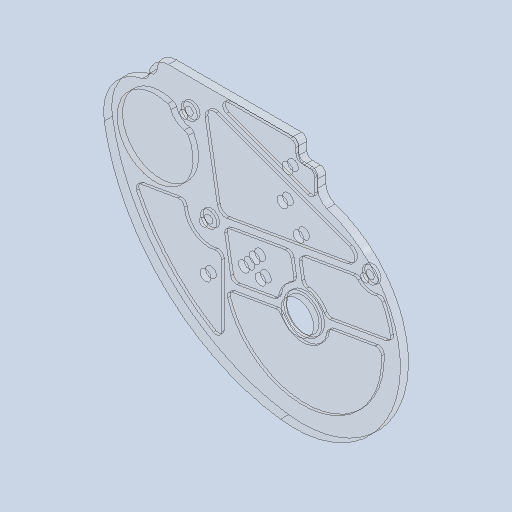
# Autodesk Inventor part: 足外フレーム
Saved by Autodesk Inventor 2023 (Build 270158000, 158)
## iProperties
Created: 2022-01-10
Part Number: 足外フレーム
Material: Polycarbonate, Clear
Document SubType Name: Modeling
Designer: acps
Density: 1.2 g/cm^3
Appearance: Polycarbonate - Clear
Author: acps
Autodesk Inventor part; units mm, degrees
ref_plane "YZ Plane" through (0, 0, 0) normal (1, 0, 0) x (0, 1, 0)
ref_plane "XZ Plane" through (0, 0, 0) normal (0, 1, 0) x (-1, 0, 0)
ref_plane "XY Plane" through (0, 0, 0) normal (0, 0, 1) x (1, 0, 0)
sketch "Sketch6" plane through (0, 0, 0) normal (0, 0, 1) x (1, 0, 0)
  circle A0 centre (46.616, 30) radius 14 construction
  circle A1 centre (67.0906, 21) radius 20.5 construction
  circle A2 centre (100, 0) radius 30 construction
  arc A3 (42.888, 47.6097) -> (28.8684, 26.9964) centre (46.616, 30) ccw
  arc A4 (93.8028, -35.6609) -> (110.9454, 40.1044) centre (98.9344, 3) ccw
  arc A5 (28.8684, 26.9964) -> (93.8028, -35.6609) centre (103.8028, 39.6783) ccw
  line L0 (-13.9923, -60) -> (152.4896, -60) construction
  arc A6 (131.1289, 13.9322) -> (113.2981, 33.8169) centre (98.9344, 3) ccw construction
  circle A7 centre (124.8574, 25) radius 3
  circle A8 centre (58.1571, 43.8132) radius 3
  circle A9 centre (65.359, 13) radius 3
  circle A10 centre (58.1571, 43.8132) radius 4 construction
  arc A11 (42.888, 47.6097) -> (45.3636, 50.3845) centre (42.2376, 50.6816) ccw
  arc A12 (52.4852, 56.8614) -> (45.3636, 50.3845) centre (52.4852, 49.7076) ccw
  line L1 (78.7064, -36) -> (126.3698, -36) construction
  circle A13 centre (58.1571, 43.8132) radius 1.5
  circle A14 centre (65.359, 13) radius 1.5
  circle A15 centre (100, 0) radius 6.025
  circle A16 centre (124.8574, 25) radius 1.5
  arc A17 (68.0566, 48.172) -> (64.0683, 44.8413) centre (67.024, 45.3553) ccw
  line L2 (64.0683, 44.8413) -> (68.5525, 19.0577)
  arc A18 (68.5525, 19.0577) -> (72.0221, 16.6161) centre (71.5081, 19.5718) ccw
  arc A19 (116.6805, 24.3829) -> (117.1992, 30.1552) centre (116.1665, 27.3385) ccw
  line L3 (72.0221, 16.6161) -> (116.6805, 24.3829)
  circle A20 centre (124.8574, 25) radius 6 construction
  circle A21 centre (58.1571, 43.8132) radius 6 construction
  circle A22 centre (65.359, 13) radius 6 construction
  line L4 (68.0566, 48.172) -> (117.1992, 30.1552)
  line L5 (72.9191, 13.7271) -> (93.4394, 17.2959)
  arc A23 (95.7525, 15.6682) -> (93.4394, 17.2959) centre (93.7821, 15.3255) ccw
  line L6 (95.7525, 15.6682) -> (96.7308, 10.0431)
  arc A24 (95.7109, 7.9407) -> (96.7308, 10.0431) centre (94.7604, 9.7004) ccw
  arc A25 (95.7109, 7.9407) -> (91.0775, 1.3563) centre (100, 0) ccw
  arc A26 (89.4429, -0.3135) -> (91.0775, 1.3563) centre (89.1002, 1.6569) ccw
  line L7 (75.7744, -2.6907) -> (89.4429, -0.3135)
  line L8 (100, 0) -> (96.3736, 20.8512) construction
  arc A27 (72.9191, 13.7271) -> (71.2914, 11.414) centre (73.2618, 11.7567) ccw
  line L9 (71.2914, 11.414) -> (73.4613, -1.063)
  arc A28 (73.4613, -1.063) -> (75.7744, -2.6907) centre (75.4317, -0.7203) ccw
  line L10 (129.5563, 5.1403) -> (73.9605, -4.5287) construction
  arc A29 (100.3359, 18.4953) -> (98.7082, 16.1822) centre (100.6786, 16.5249) ccw
  line L11 (98.7082, 16.1822) -> (99.6865, 10.5571)
  arc A30 (99.6865, 10.5571) -> (101.3563, 8.9225) centre (101.6569, 10.8998) ccw
  line L12 (100.3359, 18.4953) -> (118.5316, 21.6598)
  arc A31 (120.3701, 21.017) -> (118.5316, 21.6598) centre (118.8743, 19.6894) ccw
  arc A32 (107.9407, 4.2891) -> (101.3563, 8.9225) centre (100, 0) ccw
  arc A33 (107.9407, 4.2891) -> (110.0431, 3.2692) centre (109.7004, 5.2396) ccw
  line L13 (110.0431, 3.2692) -> (130.7399, 6.8687)
  arc A34 (130.7399, 6.8687) -> (132.3636, 9.204) centre (130.3972, 8.8391) ccw
  arc A35 (120.3701, 21.017) -> (126.8308, 19.3338) centre (124.8574, 25) ccw
  arc A36 (129.2732, 18.3479) -> (126.8308, 19.3338) centre (127.4886, 17.4451) ccw
  arc A37 (132.3636, 9.204) -> (129.2732, 18.3479) centre (98.9344, 3) ccw
  arc A38 (92.0593, -4.2891) -> (108.9225, -1.3563) centre (100, 0) ccw
  arc A39 (92.0593, -4.2891) -> (89.9569, -3.2692) centre (90.2996, -5.2396) ccw
  arc A40 (110.5571, 0.3135) -> (108.9225, -1.3563) centre (110.8998, -1.6569) ccw
  line L14 (110.5571, 0.3135) -> (126.6581, 3.1137)
  line L15 (89.9569, -3.2692) -> (73.8559, -6.0694)
  arc A41 (73.8559, -6.0694) -> (72.2892, -8.6348) centre (74.1986, -8.0398) ccw
  arc A42 (128.999, 1.2279) -> (126.6581, 3.1137) centre (127.0008, 1.1433) ccw
  arc A43 (72.2892, -8.6348) -> (128.999, 1.2279) centre (100, 0) ccw
  arc A44 (51.2056, 43.2263) -> (58.8155, 36.8682) centre (46.616, 30) ccw
  arc A45 (52.4518, 41.9559) -> (51.2056, 43.2263) centre (50.55, 41.3368) ccw
  arc A46 (58.8155, 36.8682) -> (57.3438, 37.8686) centre (57.0728, 35.887) ccw
  arc A47 (52.4518, 41.9559) -> (57.3438, 37.8686) centre (58.1571, 43.8132) ccw
  arc A48 (38.758, 8.8048) -> (67.0654, -22.2439) centre (103.8028, 39.6783) ccw
  arc A49 (40.2222, 11.6328) -> (38.758, 8.8048) centre (40.5648, 9.6624) ccw
  line L16 (40.2222, 11.6328) -> (54.0558, 14.0387)
  arc A50 (56.3913, 12.2377) -> (54.0558, 14.0387) centre (54.3985, 12.0683) ccw
  arc A51 (56.3913, 12.2377) -> (67.5901, 4.2809) centre (65.359, 13) ccw
  arc A52 (70.0859, 2.3434) -> (67.5901, 4.2809) centre (68.0859, 2.3434) ccw
  line L17 (70.0859, 2.3434) -> (70.0859, -20.5239)
  arc A53 (67.0654, -22.2439) -> (70.0859, -20.5239) centre (68.0859, -20.5239) ccw
  arc A54 (34.4673, 18.1085) -> (59.1679, 18.5348) centre (46.616, 30) ccw construction
  line L18 (52.4852, 56.8614) -> (98.4852, 56.8614)
  arc A55 (100.4852, 54.8614) -> (98.4852, 56.8614) centre (98.4852, 54.8614) ccw
  line L19 (100.4852, 54.8614) -> (100.4852, 51.8614)
  arc A56 (100.4852, 51.8614) -> (102.4852, 49.8614) centre (102.4852, 51.8614) ccw
  line L20 (102.4852, 49.8614) -> (105.4852, 49.8614)
  arc A57 (107.4852, 47.8614) -> (105.4852, 49.8614) centre (105.4852, 47.8614) ccw
  line L21 (107.4852, 47.8614) -> (107.4852, 44.8614)
  arc A58 (107.4852, 44.8614) -> (110.9454, 40.1044) centre (112.4852, 44.8614) ccw
  line L22 (71.8306, 49.9836) -> (101.7968, 38.9973)
  arc A59 (72.5191, 53.8614) -> (71.8306, 49.9836) centre (72.5191, 51.8614) ccw
  line L23 (72.5191, 53.8614) -> (95.4852, 53.8614)
  arc A60 (97.4852, 51.8614) -> (95.4852, 53.8614) centre (95.4852, 51.8614) ccw
  line L24 (97.4852, 51.8614) -> (97.4852, 49.8614)
  arc A61 (97.4852, 49.8614) -> (99.4852, 47.8614) centre (99.4852, 49.8614) ccw
  line L25 (99.4852, 47.8614) -> (102.4852, 47.8614)
  arc A62 (104.4852, 45.8614) -> (102.4852, 47.8614) centre (102.4852, 45.8614) ccw
  line L26 (104.4852, 45.8614) -> (104.4852, 40.8751)
  arc A63 (101.7968, 38.9973) -> (104.4852, 40.8751) centre (102.4852, 40.8751) ccw
  circle A64 centre (100, 0) radius 7.025
  circle A65 centre (84.2988, 11.1193) radius 3 construction
  circle A66 centre (80.3175, 6.3665) radius 3 construction
  circle A67 centre (86.4242, 5.295) radius 3 construction
  circle A68 centre (94.5653, 34.0473) radius 3.525 construction
  circle A69 centre (100.4873, 25.9894) radius 2.85 construction
  circle A70 centre (84.2988, 11.1193) radius 2
  circle A71 centre (80.3175, 6.3665) radius 2
  circle A72 centre (86.4242, 5.295) radius 2
  circle A73 centre (94.5653, 34.0473) radius 2
  circle A74 centre (100.4873, 25.9894) radius 2
  circle A75 centre (66.1789, -3.483) radius 3 construction
  circle A76 centre (66.1789, -3.483) radius 2
  circle A77 centre (96.3994, 45.7756) radius 1.25 construction
  circle A78 centre (96.3994, 45.7756) radius 2
  point P0 (0, 0)
  point P1 (100, 0)
  point P2 (44.5807, 48.5912)
  point P3 (47.672, 55)
  point P4 (132.0393, 7.6974)
  dimension "d196" = 4
  dimension "d197" = 60
  dimension "d198" = 76
  dimension "d199" = 39
  dimension "d200" = 5
  dimension "d201" = 6
  dimension "d202" = 6
  dimension "d203" = 25
  dimension "d204" = 6
  dimension "d205" = 37
  dimension "d206" = 13
  dimension "d207" = 1
  dimension "d208" = 3.14
  dimension "d209" = 48.5912
  dimension "d210" = 42.888
  dimension "d211" = 24
  dimension "d212" = 3
  dimension "d213" = 3
  dimension "d214" = 12.05
  dimension "d215" = 3
  dimension "d216" = 3
  dimension "d217" = 3
  dimension "d218" = 3
  dimension "d219" = 3
  dimension "d220" = 3
  dimension "d221" = 3
  dimension "d222" = 30
  dimension "d223" = 90
  dimension "d224" = 2
  dimension "d225" = 2
  dimension "d226" = 3
  dimension "d227" = 2
  dimension "d228" = 2
  dimension "d229" = 2
  dimension "d230" = 3
  dimension "d231" = 1.5
  dimension "d232" = 1.5
  dimension "d233" = 2
  dimension "d234" = 2
  dimension "d235" = 2
  dimension "d236" = 3
  dimension "d237" = 1.5
  dimension "d238" = 3
  dimension "d239" = 2
  dimension "d240" = 1.5
  dimension "d241" = 2
  dimension "d242" = 2
  dimension "d243" = 2
  dimension "d244" = 2
  dimension "d245" = 3
  dimension "d246" = 1.5
  dimension "d247" = 1.5
  dimension "d248" = 2
  dimension "d249" = 2
  dimension "d250" = 20
  dimension "d251" = 2
  dimension "d252" = 2
  dimension "d253" = 2
  dimension "d254" = 4
  dimension "d255" = 2
  dimension "d256" = 2
  dimension "d257" = 2
  dimension "d258" = 3
  dimension "d259" = 3
  constraints: 109 point on circle, 82 tangent, 78 centre point, 54 end point, 13 concentric, 12 coincident, 11 parallel, 6 horizontal, 6 vertical, 2 perpendicular, 2 point on line, 25 other
  measures "d196" radial gap between concentric circles of A0 A3
  measures "d197" distance from line of L0 point (0, 0)
  measures "d198" radius of A5
  measures "d199" radius of A4
  measures "d200" radial gap between concentric circles of A4 A6
  measures "d201" diameter of A7
  measures "d202" diameter of A8
  measures "d203" vertical distance of point (0, 0) A7.centre
  measures "d204" diameter of A9
  measures "d205" distance of point (100, 0) A9.centre
  measures "d206" vertical distance of point (0, 0) A9.centre
  measures "d207" radial gap between concentric circles of A8 A10
  measures "d208" radius of A11
  measures "d209" vertical distance of point (0, 0) point (44.581, 48.591)
  measures "d210" horizontal distance of point (0, 0) A3.start
  measures "d211" distance between parallel lines of L0 L1
  measures "d212" diameter of A13
  measures "d213" diameter of A14
  measures "d214" diameter of A15
  measures "d215" diameter of A16
  measures "d216" radius of A17
  measures "d217" radius of A18
  measures "d218" radius of A19
  measures "d219" radial gap between concentric circles of A7 A20
  measures "d220" radial gap between concentric circles of A8 A21
  measures "d221" radial gap between concentric circles of A9 A22
  measures "d222" angle of L3 L4
  measures "d223" angle of L3 L2
  measures "d224" radius of A23
  measures "d225" radius of A24
  measures "d226" radial gap between concentric circles of A15 A25
  measures "d227" radius of A26
  measures "d228" radius of A27
  measures "d229" radius of A28
  measures "d230" distance between parallel lines of L3 L5
  measures "d231" distance between parallel lines of L8 L6
  measures "d232" distance between parallel lines of L10 L7
  measures "d233" radius of A29
  measures "d234" radius of A30
  measures "d235" radius of A31
  measures "d236" distance between parallel lines of L12 L3
  measures "d237" distance between parallel lines of L8 L11
  measures "d238" radial gap between concentric circles of A15 A32
  measures "d239" radius of A33
  measures "d240" distance between parallel lines of L10 L13
  measures "d241" radius of A34
  measures "d242" radius of A36
  measures "d243" radius of A39
  measures "d244" radius of A40
  measures "d245" radial gap between concentric circles of A38 A15
  measures "d246" distance between parallel lines of L15 L10
  measures "d247" distance between parallel lines of L10 L14
  measures "d248" radius of A41
  measures "d249" radius of A42
  measures "d250" radial gap between concentric circles of A43 A38
  measures "d251" radius of A45
  measures "d252" radius of A46
  measures "d253" radius of A49
  measures "d254" radial gap between concentric circles of A5 A48
  measures "d255" radius of A50
  measures "d256" radius of A52
  measures "d257" radius of A53
  measures "d258" radial gap between concentric circles of A22 A51
  measures "d259" radial gap between concentric circles of A54 A0
extrude "Extrusion4" add sketch "Sketch6" along normal blind 3 contours A11 A12 L18 A55 L19 A56 L20 A57 L21 A58 A4 A5 A3 | A7 | A8 | A9 | L4 A19 L3 A18 L2 A17 | L5 A23 L6 A24 A25 A26 L7 A28 L9 A27 | L12 A31 A35 A36 A37 A34 L13 A33 A32 A30 L11 A29 | A38 A40 L14 A42 A43 A41 L15 A39 | A45 A47 A46 A44 | A49 L16 A50 A51 A52 L17 A53 A48 | A59 L23 A60 L24 A61 L25 A62 L26 A63 L22 | A64
sketch "Sketch10" plane through (0, 0, 0) normal (0, 0, -1) x (-1, 0, 0)
  line L0 (-68.0566, 48.172) -> (-117.1992, 30.1552) projected
  arc A0 (-117.1992, 30.1552) -> (-116.6805, 24.3829) centre (-116.1665, 27.3385) ccw projected
  line L1 (-72.0221, 16.6161) -> (-116.6805, 24.3829) projected
  arc A1 (-72.0221, 16.6161) -> (-68.5525, 19.0577) centre (-71.5081, 19.5718) ccw projected
  line L2 (-64.0683, 44.8413) -> (-68.5525, 19.0577) projected
  arc A2 (-57.3438, 37.8686) -> (-52.4518, 41.9559) centre (-58.1571, 43.8132) ccw projected
  circle A3 centre (-58.1571, 43.8132) radius 3 projected
  circle A4 centre (-124.8574, 25) radius 3 projected
  circle A5 centre (-65.359, 13) radius 3 projected
  line L3 (-100.3359, 18.4953) -> (-118.5316, 21.6598) projected
  arc A6 (-118.5316, 21.6598) -> (-120.3701, 21.017) centre (-118.8743, 19.6894) ccw projected
  arc A7 (-126.8308, 19.3338) -> (-120.3701, 21.017) centre (-124.8574, 25) ccw projected
  arc A8 (-126.8308, 19.3338) -> (-129.2732, 18.3479) centre (-127.4886, 17.4451) ccw projected
  arc A9 (-129.2732, 18.3479) -> (-132.3636, 9.204) centre (-98.9344, 3) ccw projected
  arc A10 (-132.3636, 9.204) -> (-130.7399, 6.8687) centre (-130.3972, 8.8391) ccw projected
  line L4 (-110.0431, 3.2692) -> (-130.7399, 6.8687) projected
  arc A11 (-110.0431, 3.2692) -> (-107.9407, 4.2891) centre (-109.7004, 5.2396) ccw projected
  arc A12 (-101.3563, 8.9225) -> (-107.9407, 4.2891) centre (-100, 0) ccw projected
  arc A13 (-101.3563, 8.9225) -> (-99.6865, 10.5571) centre (-101.6569, 10.8998) ccw projected
  line L5 (-98.7082, 16.1822) -> (-99.6865, 10.5571) projected
  arc A14 (-98.7082, 16.1822) -> (-100.3359, 18.4953) centre (-100.6786, 16.5249) ccw projected
  arc A15 (-91.0775, 1.3563) -> (-95.7109, 7.9407) centre (-100, 0) ccw projected
  arc A16 (-96.7308, 10.0431) -> (-95.7109, 7.9407) centre (-94.7604, 9.7004) ccw projected
  line L6 (-95.7525, 15.6682) -> (-96.7308, 10.0431) projected
  arc A17 (-93.4394, 17.2959) -> (-95.7525, 15.6682) centre (-93.7821, 15.3255) ccw projected
  line L7 (-72.9191, 13.7271) -> (-93.4394, 17.2959) projected
  arc A18 (-71.2914, 11.414) -> (-72.9191, 13.7271) centre (-73.2618, 11.7567) ccw projected
  line L8 (-71.2914, 11.414) -> (-73.4613, -1.063) projected
  arc A19 (-75.7744, -2.6907) -> (-73.4613, -1.063) centre (-75.4317, -0.7203) ccw projected
  line L9 (-75.7744, -2.6907) -> (-89.4429, -0.3135) projected
  arc A20 (-91.0775, 1.3563) -> (-89.4429, -0.3135) centre (-89.1002, 1.6569) ccw projected
  line L10 (-110.5571, 0.3135) -> (-126.6581, 3.1137) projected
  arc A21 (-108.9225, -1.3563) -> (-110.5571, 0.3135) centre (-110.8998, -1.6569) ccw projected
  arc A22 (-126.6581, 3.1137) -> (-128.999, 1.2279) centre (-127.0008, 1.1433) ccw projected
  arc A23 (-128.999, 1.2279) -> (-72.2892, -8.6348) centre (-100, 0) ccw projected
  arc A24 (-108.9225, -1.3563) -> (-92.0593, -4.2891) centre (-100, 0) ccw projected
  arc A25 (-89.9569, -3.2692) -> (-92.0593, -4.2891) centre (-90.2996, -5.2396) ccw projected
  line L11 (-89.9569, -3.2692) -> (-73.8559, -6.0694) projected
  arc A26 (-72.2892, -8.6348) -> (-73.8559, -6.0694) centre (-74.1986, -8.0398) ccw projected
  arc A27 (-67.0654, -22.2439) -> (-38.758, 8.8048) centre (-103.8028, 39.6783) ccw projected
  arc A28 (-70.0859, -20.5239) -> (-67.0654, -22.2439) centre (-68.0859, -20.5239) ccw projected
  line L12 (-70.0859, 2.3434) -> (-70.0859, -20.5239) projected
  arc A29 (-67.5901, 4.2809) -> (-70.0859, 2.3434) centre (-68.0859, 2.3434) ccw projected
  arc A30 (-67.5901, 4.2809) -> (-56.3913, 12.2377) centre (-65.359, 13) ccw projected
  arc A31 (-54.0558, 14.0387) -> (-56.3913, 12.2377) centre (-54.3985, 12.0683) ccw projected
  line L13 (-40.2222, 11.6328) -> (-54.0558, 14.0387) projected
  arc A32 (-38.758, 8.8048) -> (-40.2222, 11.6328) centre (-40.5648, 9.6624) ccw projected
  arc A33 (-99.4852, 47.8614) -> (-97.4852, 49.8614) centre (-99.4852, 49.8614) ccw projected
  line L14 (-99.4852, 47.8614) -> (-102.4852, 47.8614) projected
  arc A34 (-102.4852, 47.8614) -> (-104.4852, 45.8614) centre (-102.4852, 45.8614) ccw projected
  line L15 (-104.4852, 45.8614) -> (-104.4852, 40.8751) projected
  arc A35 (-104.4852, 40.8751) -> (-101.7968, 38.9973) centre (-102.4852, 40.8751) ccw projected
  line L16 (-71.8306, 49.9836) -> (-101.7968, 38.9973) projected
  arc A36 (-71.8306, 49.9836) -> (-72.5191, 53.8614) centre (-72.5191, 51.8614) ccw projected
  line L17 (-72.5191, 53.8614) -> (-95.4852, 53.8614) projected
  arc A37 (-95.4852, 53.8614) -> (-97.4852, 51.8614) centre (-95.4852, 51.8614) ccw projected
  line L18 (-97.4852, 51.8614) -> (-97.4852, 49.8614) projected
  arc A38 (-58.8155, 36.8682) -> (-51.2056, 43.2263) centre (-46.616, 30) ccw projected
  circle A39 centre (-46.616, 30) radius 14 construction
  arc A40 (-57.3438, 37.8686) -> (-58.8155, 36.8682) centre (-57.0728, 35.887) ccw projected
  arc A41 (-51.2056, 43.2263) -> (-52.4518, 41.9559) centre (-50.55, 41.3368) ccw projected
  point P0 (0, 0)
extrude "Extrusion9" cut sketch "Sketch6" along normal blind 1 contours A7 | A8 | A9 | L4 A19 L3 A18 L2 A17 | L5 A23 L6 A24 A25 A26 L7 A28 L9 A27 | L12 A31 A35 A36 A37 A34 L13 A33 A32 A30 L11 A29 | A38 A40 L14 A42 A43 A41 L15 A39 | A49 L16 A50 A51 A52 L17 A53 A48 | A59 L23 A60 L24 A61 L25 A62 L26 A63 L22 | A64 | A70 | A71 | A72 | A73 | A74 | A76 | A78
extrude "Extrusion11" cut sketch "Sketch6" along normal blind 2 contours A45 A47 A46 A44
body "Solid2"
